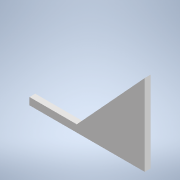
# Autodesk Inventor part: Part3
Saved by Autodesk Inventor 2021 (Build 250183000, 183)
## iProperties
Created: 2020-07-15
Part Number: Part3
Material: Generic
Document SubType Name: Modeling
Designer: adick
Density: 1 g/cm^3
Appearance: Default
Author: adick
Autodesk Inventor part; units mm, degrees
ref_plane "YZ Plane" through (0, 0, 0) normal (1, 0, 0) x (0, 1, 0)
ref_plane "XZ Plane" through (0, 0, 0) normal (0, 1, 0) x (-1, 0, 0)
ref_plane "XY Plane" through (0, 0, 0) normal (0, 0, 1) x (1, 0, 0)
sketch "Sketch1" plane through (0, 0, 0) normal (0, 0, 1) x (1, 0, 0)
  line L0 (252.3, 12.7) -> (0.0018, 12.7)
  line L1 (0.0018, 12.7) -> (0.0018, 28.399)
  line L2 (0.0018, 28.399) -> (103.5611, 28.399)
  line L3 (252.3, 28.399) -> (252.3, 12.7)
  line L4 (252.3, 190.5) -> (103.5611, 28.399)
  line L5 (252.3, 28.399) -> (252.3, 190.5)
  point P0 (0, 0)
  point P1 (0, 12.7)
  dimension "d2" = 220
  constraints: 12 end point, 2 parallel, 1 horizontal, 1 perpendicular, 1 point on line, 1 vertical, 3 other
  measures "d2" distance of L2.end L4.start
extrude "Extrusion1" add sketch "Sketch1" against normal blind 12.7
body "Solid1"
